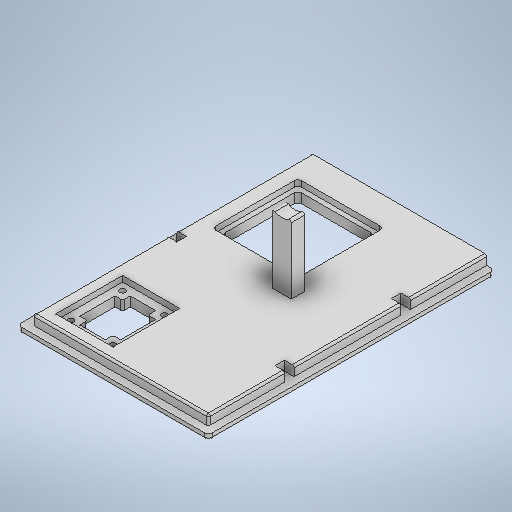
# Autodesk Inventor part: body-1
Saved by Autodesk Inventor 2025 (Build 290162000, 162)
## iProperties
Created: 2026-01-27
Part Number: body-1
Material: 一般
Document SubType Name: Modeling
Designer: mahhy
Density: 1 g/cm^3
Appearance: 既定
Author: mahhy
## iProperties of the stored document body-1_3D プリント.ipt
Created: 2026-01-28
Part Number: body-1_3D プリント
Material: 一般
Document SubType Name: Modeling
Designer: mahhy
Density: 1 g/cm^3
Appearance: 既定
Author: mahhy
Autodesk Inventor part; units mm, degrees
ref_plane "YZ Plane" through (0, 0, 0) normal (1, 0, 0) x (0, 1, 0)
ref_plane "XZ Plane" through (0, 0, 0) normal (0, 1, 0) x (-1, 0, 0)
ref_plane "XY Plane" through (0, 0, 0) normal (0, 0, 1) x (1, 0, 0)
sketch "底面スケッチ" plane through (0, 0, 0) normal (0, 1, 0) x (-1, 0, 0)
  line L0 (0, 0) -> (100, 0)
  line L1 (100, 0) -> (100, -150)
  line L2 (100, -150) -> (0, -150)
  line L3 (0, -150) -> (0, 0)
  line L4 (83.5, -92.5) -> (47.5, -92.5)
  line L5 (45.5, -94.5) -> (45.5, -130.5)
  line L6 (47.5, -132.5) -> (83.5, -132.5)
  line L7 (85.5, -130.5) -> (85.5, -94.5)
  arc A0 (85.5, -94.5) -> (83.5, -92.5) centre (83.5, -94.5) ccw
  arc A1 (83.5, -132.5) -> (85.5, -130.5) centre (83.5, -130.5) ccw
  arc A2 (45.5, -130.5) -> (47.5, -132.5) centre (47.5, -130.5) ccw
  arc A3 (47.5, -92.5) -> (45.5, -94.5) centre (47.5, -94.5) ccw
  point P0 (85.5, -92.5)
  point P1 (45.5, -132.5)
  point P2 (45.5, -92.5)
  point P3 (85.5, -132.5)
  dimension "d0" = 100
  dimension "d1" = 150
  dimension "d34" = 40
  dimension "d38" = 2
  dimension "d40" = 40
  dimension "d41" = 14.5
  dimension "d49" = 92.5
  constraints: 16 end point, 8 point on circle, 8 point on line, 8 tangent, 4 centre point, 4 parallel, 3 equal radius, 2 horizontal, 2 perpendicular
  measures "d0" distance of L1.end L2.end
  measures "d1" distance of L0.end L1.end
  measures "d34" distance of point (85.5, -132.5) point (45.5, -132.5)
  measures "d38" radius of A0
  measures "d40" distance between parallel lines of L6 L4
  measures "d41" distance between parallel lines of L1 L7
  measures "d49" distance between parallel lines of L0 L4
extrude "底面" add sketch "底面スケッチ" along normal blind 8
sketch "スケッチ2" plane through (0, 8, 0) normal (0, 1, 0) x (1, 0, 0)
  line L0 (-90, 10) -> (-60, 10)
  line L1 (-60, 10) -> (-60, 45)
  line L2 (-60, 45) -> (-90, 45)
  line L3 (-90, 45) -> (-90, 10)
  line L4 (-100, 0) -> (0, 0) projected
  line L5 (-100, 150) -> (-100, 0) projected
  dimension "d12" = 30
  dimension "d13" = 35
  dimension "d15" = 10
  dimension "d50" = 10
  constraints: 8 end point, 2 parallel, 1 horizontal, 1 perpendicular
  measures "d12" distance of L2.end L1.end
  measures "d13" distance of L1.end L0.end
  measures "d15" distance between parallel lines of L5 L3
  measures "d50" distance between parallel lines of L4 L0
extrude "溝" cut sketch "スケッチ2" against normal blind 3
sketch "スケッチ3" plane through (0, 8, 0) normal (0, 1, 0) x (1, 0, 0)
  line L0 (0, 0) -> (0, 150) projected
  line L1 (-100, 0) -> (0, 0) projected
  line L2 (-45, 85.5) -> (-35, 85.5)
  line L3 (-35, 85.5) -> (-35, 78.5)
  line L4 (-35, 78.5) -> (-45, 78.5)
  line L5 (-45, 78.5) -> (-45, 85.5)
  line L6 (-100, 150) -> (-100, 0) projected
  point P0 (-45, 82)
  point P1 (0, 78.5)
  point P2 (0, 85.5)
  dimension "d42" = 10
  dimension "d43" = 7
  dimension "d44" = 55
  dimension "d45" = 82
  constraints: 8 end point, 2 parallel, 1 horizontal, 1 midpoint, 1 perpendicular
  measures "d42" distance of L3.end L4.end
  measures "d43" distance of L2.end L3.end
  measures "d44" distance between parallel lines of L6 L5
  measures "d45" distance from line of L1 point (-45, 82)
extrude "支柱" add sketch "スケッチ3" along normal blind 41
sketch "スケッチ4" plane through (0, 8, -85.5) normal (0, 0, -1) x (-1, 0, 0)
  circle A0 centre (40, 41) radius 6.5
  line L0 (35, 41) -> (45, 41) projected
  point P0 (0, -8)
  dimension "d25" = 13
  constraints: 1 centre point, 1 coincident, 1 midpoint
  measures "d25" diameter of A0
extrude "押し出し4" cut sketch "スケッチ4" against normal blind 39
fillet "フィレット1" radius 1 2 edges at (-45, 44.8467, -82) (-35, 44.8467, -82)
sketch "スケッチ5" plane through (0, 8, 0) normal (0, 1, 0) x (1, 0, 0)
  line L0 (-86, 90) -> (-45, 90)
  line L1 (-43, 92) -> (-43, 133)
  line L2 (-45, 135) -> (-86, 135)
  line L3 (-88, 133) -> (-88, 92)
  line L4 (0, 150) -> (-100, 150) projected
  line L5 (0, 0) -> (0, 150) projected
  arc A0 (-88, 92) -> (-86, 90) centre (-86, 92) ccw
  arc A1 (-86, 135) -> (-88, 133) centre (-86, 133) ccw
  arc A2 (-43, 133) -> (-45, 135) centre (-45, 133) ccw
  arc A3 (-45, 90) -> (-43, 92) centre (-45, 92) ccw
  line L6 (-100, 150) -> (-100, 0) projected
  line L7 (-100, 0) -> (0, 0) projected
  point P0 (-88, 90)
  point P1 (-43, 135)
  point P2 (-43, 90)
  point P3 (-88, 135)
  point P4 (0, 85.5)
  dimension "d27" = 45
  dimension "d28" = 45
  dimension "d33" = 2
  dimension "d46" = 12
  dimension "d51" = 90
  constraints: 8 end point, 8 point on circle, 8 point on line, 8 tangent, 4 centre point, 3 equal radius, 2 parallel, 1 horizontal, 1 perpendicular
  measures "d27" distance of point (-88, 135) point (-43, 135)
  measures "d28" distance of point (-43, 90) point (-43, 135)
  measures "d33" radius of A0
  measures "d46" distance between parallel lines of L6 L3
  measures "d51" distance between parallel lines of L7 L0
extrude "ケース用溝" cut sketch "スケッチ5" against normal blind 3 contours A0 L3 A1 L2 A2 L1 A3 L0
fillet "フィレット2" radius 2 4 edges at (0, 4, 0) (-100, 4, 0) (0, 4, -150) (-100, 4, -150)
fillet "フィレット3" radius 1 8 edges at (-0.5858, 0, -149.4142) (-50, 0, -150) (-99.4142, 0, -149.4142) (-100, 0, -75) (-99.4142, 0, -0.5858) (-50, 0, 0) (-0.5858, 0, -0.5858) (0, 0, -75)
sketch "スケッチ6" plane through (0, 8, 0) normal (0, 1, 0) x (1, 0, 0)
  line L0 (-96, 150) -> (-4, 150)
  line L1 (-4, 150) -> (-4, 4)
  line L2 (-4, 4) -> (-96, 4)
  line L3 (-96, 4) -> (-96, 150)
  line L4 (-100, 148) -> (-100, 2) projected
  line L5 (-2, 150) -> (-98, 150) projected
  line L6 (0, 2) -> (0, 148) projected
  line L7 (-98, 0) -> (-2, 0) projected
  arc A0 (-2, 0) -> (0, 2) centre (-2, 2) ccw projected
  arc A1 (-100, 2) -> (-98, 0) centre (-98, 2) ccw projected
  arc A2 (0, 148) -> (-2, 150) centre (-2, 148) ccw projected
  arc A3 (-98, 150) -> (-100, 148) centre (-98, 148) ccw projected
  line L8 (-4, 44) -> (-9, 44)
  line L9 (-9, 44) -> (-9, 49)
  line L10 (-9, 49) -> (-4, 49)
  line L11 (-4, 49) -> (-4, 44)
  line L12 (-4, 105) -> (-9, 105)
  line L13 (-9, 105) -> (-9, 110)
  line L14 (-9, 110) -> (-4, 110)
  line L15 (-4, 110) -> (-4, 105)
  line L16 (-96, 74.5) -> (-91, 74.5)
  line L17 (-91, 74.5) -> (-91, 79.5)
  line L18 (-91, 79.5) -> (-96, 79.5)
  line L19 (-96, 79.5) -> (-96, 74.5)
  point P0 (0, 0)
  point P1 (-96, 77)
  point P2 (-96, 77)
  point P3 (-4, 110)
  dimension "d54" = 4
  dimension "d56" = 4
  dimension "d57" = 4
  dimension "d60" = 5
  dimension "d62" = 40
  dimension "d63" = 5
  dimension "d64" = 5
  dimension "d65" = 5
  dimension "d66" = 40
  dimension "d67" = 5
  dimension "d68" = 5
  dimension "d100" = 0
  constraints: 32 end point, 8 parallel, 4 horizontal, 4 perpendicular, 3 point on line, 2 midpoint, 1 coincident
  measures "d54" distance between parallel lines of L4 L3
  measures "d56" distance between parallel lines of L6 L1
  measures "d57" distance between parallel lines of L7 L2
  measures "d60" distance of L8.end L9.end
  measures "d62" distance from line of L8.start L2
  measures "d63" distance of L8.start L8.end
  measures "d64" distance of L12.end L13.end
  measures "d65" distance of L13.end L14.end
  measures "d66" distance between parallel lines of L0 L14
  measures "d67" distance of L18.end L17.end
  measures "d68" distance of L17.end L16.end
  measures "d100" distance between parallel lines of L5 L0
extrude "押し出し6" cut sketch "スケッチ6" against normal blind 5 contours L3 L2 L1 L5 A2 L6 A0 L7 A1 L4 A3 | L18 L17 L16 L3 | L1 L12 L13 L14 | L1 L8 L9 L10
sketch "スケッチ7" plane through (0, 5, 0) normal (0, 1, 0) x (1, 0, 0)
  circle A0 centre (-86, 14) radius 1.5
  circle A1 centre (-64, 14) radius 1.5
  circle A2 centre (-86, 41) radius 1.5
  circle A3 centre (-64, 41) radius 1.5
  line L0 (-90, 45) -> (-60, 45) projected
  line L1 (-60, 10) -> (-90, 10) projected
  line L2 (-90, 10) -> (-90, 45) projected
  line L3 (-60, 45) -> (-60, 10) projected
  line L4 (-85.7, 18.3) -> (-64.3, 18.3)
  line L5 (-64.3, 18.3) -> (-64.3, 36.7)
  line L6 (-64.3, 36.7) -> (-85.7, 36.7)
  line L7 (-85.7, 36.7) -> (-85.7, 18.3)
  line L8 (-81.7, 14.3) -> (-68.3, 14.3)
  line L9 (-68.3, 14.3) -> (-68.3, 40.7)
  line L10 (-68.3, 40.7) -> (-81.7, 40.7)
  line L11 (-81.7, 40.7) -> (-81.7, 14.3)
  point P0 (0, 0)
  point P1 (-81.7, 36.7)
  point P2 (-81.7, 18.3)
  point P3 (-68.3, 18.3)
  point P4 (-68.3, 36.7)
  dimension "d69" = 3
  dimension "d70" = 3
  dimension "d71" = 3
  dimension "d72" = 3
  dimension "d73" = 4
  dimension "d74" = 4
  dimension "d75" = 4
  dimension "d76" = 4
  dimension "d79" = 4.3
  dimension "d80" = 4.3
  dimension "d81" = 4.3
  dimension "d82" = 4.3
  dimension "d83" = 4.3
  dimension "d84" = 4.3
  dimension "d85" = 4.3
  dimension "d86" = 4.3
  constraints: 16 end point, 4 centre point, 4 parallel, 2 horizontal, 2 horizontal alignment, 2 perpendicular, 2 vertical alignment
  measures "d69" diameter of A0
  measures "d70" diameter of A1
  measures "d71" diameter of A2
  measures "d72" diameter of A3
  measures "d73" distance from line of L0 A2.centre
  measures "d74" distance from line of L1 A0.centre
  measures "d75" distance from line of L2 A2.centre
  measures "d76" distance from line of L3 A3.centre
  measures "d79" distance from line of A2.centre L6
  measures "d80" distance from line of A0.centre L4
  measures "d81" distance between parallel lines of L2 L7
  measures "d82" distance between parallel lines of L3 L5
  measures "d83" distance between parallel lines of L0 L10
  measures "d84" distance between parallel lines of L1 L8
  measures "d85" distance from line of L11 A2.centre
  measures "d86" distance from line of A3.centre L9
extrude "ネジ穴" cut sketch "スケッチ7" against normal through all contours A0 | A1 | A2 | A3 | L7 L6 L11 L4 | L11 L6 L9 L4 | L4 L9 L8 L11 | L9 L6 L5 L4 | L11 L10 L9 L6
fillet "フィレット4" radius 1 4 edges at (-81.7, 2.5, -18.3) (-81.7, 2.5, -36.7) (-68.3, 2.5, -36.7) (-68.3, 2.5, -18.3)
sketch "スケッチ8" plane through (0, 0, 0) normal (0, -1, 0) x (1, 0, 0)
  line L0 (-67.9, -41) -> (-65.95, -37.6225)
  line L1 (-65.95, -37.6225) -> (-62.05, -37.6225)
  line L2 (-62.05, -37.6225) -> (-60.1, -41)
  line L3 (-60.1, -41) -> (-62.05, -44.3775)
  line L4 (-62.05, -44.3775) -> (-65.95, -44.3775)
  line L5 (-65.95, -44.3775) -> (-67.9, -41)
  line L6 (-87.95, -37.6225) -> (-84.05, -37.6225)
  line L7 (-84.05, -37.6225) -> (-82.1, -41)
  line L8 (-82.1, -41) -> (-84.05, -44.3775)
  line L9 (-84.05, -44.3775) -> (-87.95, -44.3775)
  line L10 (-87.95, -44.3775) -> (-89.9, -41)
  line L11 (-89.9, -41) -> (-87.95, -37.6225)
  line L12 (-65.95, -10.6225) -> (-62.05, -10.6225)
  line L13 (-62.05, -10.6225) -> (-60.1, -14)
  line L14 (-60.1, -14) -> (-62.05, -17.3775)
  line L15 (-62.05, -17.3775) -> (-65.95, -17.3775)
  line L16 (-65.95, -17.3775) -> (-67.9, -14)
  line L17 (-67.9, -14) -> (-65.95, -10.6225)
  line L18 (-89.9, -14) -> (-87.95, -10.6225)
  line L19 (-87.95, -10.6225) -> (-84.05, -10.6225)
  line L20 (-84.05, -10.6225) -> (-82.1, -14)
  line L21 (-82.1, -14) -> (-84.05, -17.3775)
  line L22 (-84.05, -17.3775) -> (-87.95, -17.3775)
  line L23 (-87.95, -17.3775) -> (-89.9, -14)
  circle A0 centre (-86, -41) radius 1.5 projected
  circle A1 centre (-64, -14) radius 1.5 projected
  circle A2 centre (-86, -14) radius 1.5 projected
  circle A3 centre (-64, -41) radius 1.5 projected
  point P0 (0, 0)
  dimension "d95" = 3.9
  dimension "d96" = 3.9
  dimension "d97" = 3.9
  dimension "d98" = 3.9
  constraints: 48 end point, 4 coincident, 2 collinear, 52 other
  measures "d95" distance of L4.end L0.start
  measures "d96" distance of L10.end L6.start
  measures "d97" distance of L16.end L12.start
  measures "d98" distance of L22.end L18.start
extrude "ナット穴" cut sketch "スケッチ8" against normal blind 2.8 contours L0 L1 L2 L3 L4 L5 | L6 L7 L8 L9 L10 L11 | L12 L13 L14 L15 L16 L17 | L18 L19 L20 L21 L22 L23 | A3
fillet "フィレット5" radius 1 8 edges at (-4, 5.5, -4) (-96, 5.5, -4) (-96, 8, -114.75) (-96, 8, -39.25) (-4, 8, -24) (-4, 8, -77) (-4, 8, -130) (-50, 8, -4)
equation "\"d40\" = d34"
equation "\"d28\" = d27"
equation "\"d56\" = d54"
equation "\"d57\" = d54"
equation "\"d65\" = d63"
equation "\"d66\" = d62"
equation "\"d58\" = d60"
equation "\"d69\" = d71"
equation "\"d70\" = d71"
equation "\"d72\" = d71"
equation "\"d74\" = d73"
equation "\"d75\" = d73"
equation "\"d76\" = d73"
equation "\"d80\" = d79"
equation "\"d81\" = d79"
equation "\"d82\" = d79"
equation "\"d83\" = d79"
equation "\"d84\" = d79"
equation "\"d85\" = d79"
equation "\"d86\" = d79"
equation "\"d96\" = d95"
equation "\"d97\" = d95"
equation "\"d98\" = d95"
